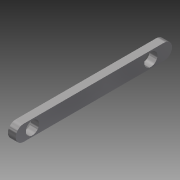
# Autodesk Inventor part: legsupport
Saved by Autodesk Inventor 2015 (Build 190159000, 159)
## iProperties
Created: 2020-01-20
Part Number: legsupport
Material: Stainless Steel, Austenitic
Document SubType Name: Modeling
Designer: hp
Density: 8 g/cm^3
Appearance: Semi-Polished
Author: hp
Autodesk Inventor part; units mm, degrees
ref_plane "YZ Plane" through (0, 0, 0) normal (1, 0, 0) x (0, 1, 0)
ref_plane "XZ Plane" through (0, 0, 0) normal (0, 1, 0) x (-1, 0, 0)
ref_plane "XY Plane" through (0, 0, 0) normal (0, 0, 1) x (1, 0, 0)
sketch "Sketch1" plane through (0, 0, 0) normal (1, 0, 0) x (0, 1, 0)
  line L0 (3.7236, 14.5672) -> (3.7236, -585.4316)
  line L1 (3.7236, -585.4316) -> (-56.2763, -585.4316)
  line L2 (-56.2763, -585.4316) -> (-56.2763, 14.5672)
  line L3 (-56.2763, 14.5672) -> (3.7236, 14.5672)
  line L4 (-26.2764, 14.5672) -> (-26.2764, -49.7456)
  circle A0 centre (-26.2764, -49.7456) radius 25.4
  line L5 (-26.2764, -585.4316) -> (-26.2764, -503.9738)
  circle A1 centre (-26.2764, -503.9738) radius 25.4
  point P0 (0, 0)
  dimension "d0" = 599.9988
  dimension "d1" = 59.9999
  dimension "d2" = 64.3128
  dimension "d3" = 50.8
  dimension "d4" = 81.4578
  dimension "d5" = 50.8
  constraints: 12 end point, 3 vertical, 2 centre point, 2 coincident, 2 midpoint, 2 perpendicular, 1 horizontal
  measures "d0" distance of L0.start L0.end
  measures "d1" distance of L0.end L1.end
  measures "d2" distance of L4.start L4.end
  measures "d3" diameter of A0
  measures "d4" distance of L5.start L5.end
  measures "d5" diameter of A1
extrude "Extrusion1" add sketch "Sketch1" along normal blind 29.9999
fillet "Fillet1" radius 30.48 4 edges at (15, 3.7236, 14.5672) (15, -56.2763, 14.5672) (15, 3.7236, -585.4316) (15, -56.2763, -585.4316)
body "Solid1"
